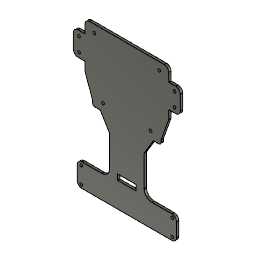
chassis (Autodesk Fusion 360 design; units mm, degrees)
part number: 2026-02-12-20-41-27-995
Autodesk Fusion 360 part; units mm, degrees
sketch "Sketch1" plane through (0, 0, 0) normal (0, 1, 0) x (1, 0, 0)
  line L0 (48.5, 0) -> (-48.5, 0)
  line L1 (-54.5, 6) -> (-54.5, 17)
  line L2 (54.5, 6) -> (54.5, 17)
  line L3 (54.5, 17) -> (54.5, 48) construction
  line L4 (-54.5, 48) -> (-54.5, 59)
  line L5 (54.5, 48) -> (54.5, 59)
  line L6 (54.4997, 87) -> (44.4997, 86.9972) construction
  line L7 (-54.5, 59) -> (-44.4997, 86.9972)
  line L8 (54.5, 59) -> (44.4997, 86.9972)
  line L9 (44.4997, 86.9972) -> (44.4989, 89.9972)
  line L10 (-44.4989, 89.9972) -> (-44.4997, 86.9972)
  line L11 (-41.498, 92.9963) -> (-34.498, 92.9943)
  line L12 (41.498, 92.9963) -> (34.498, 92.9943)
  line L13 (-34.498, 92.9943) -> (-22.5008, 113)
  line L14 (22.5008, 113) -> (34.498, 92.9943)
  line L15 (-22.5008, 113) -> (-22.5122, 153)
  line L16 (22.5008, 113) -> (22.5122, 153)
  line L17 (-32.515, 162.9972) -> (-58.515, 162.9898)
  line L18 (32.515, 162.9972) -> (58.515, 162.9898)
  line L19 (-64.5167, 168.9881) -> (-64.5219, 186.9864)
  line L20 (64.5167, 168.9881) -> (64.5219, 186.9864)
  line L21 (-58.5219, 192.9881) -> (58.5219, 192.9881)
  line L22 (-54.5, 17) -> (-63.5, 17)
  line L23 (-54.5, 48) -> (-63.5, 48)
  line L24 (-69.5, 23) -> (-69.5, 42)
  line L25 (54.5, 17) -> (63.5, 17)
  line L26 (54.5, 48) -> (63.5, 48)
  line L27 (69.5, 42) -> (69.5, 23)
  line L28 (-54.5, 0) -> (-42.1, 0) construction
  line L29 (54.5, 0) -> (42.1, 0) construction
  line L30 (54.5, 10) -> (54.5, 0) construction
  circle A0 centre (-42.1, 10) radius 1.75
  circle A1 centre (42.1, 10) radius 1.75
  circle A2 centre (-30.84, 83.28) radius 1.75
  circle A3 centre (30.84, 83.28) radius 1.75
  circle A4 centre (-62, 23.475) radius 1.75
  circle A5 centre (-62, 41.525) radius 1.75
  circle A6 centre (62, 23.475) radius 1.75
  circle A7 centre (62, 41.525) radius 1.75
  arc A8 (-54.5, 6) -> (-48.5, 0) centre (-48.5, 6) ccw
  arc A9 (48.5, 0) -> (54.5, 6) centre (48.5, 6) ccw
  arc A10 (63.5, 17) -> (69.5, 23) centre (63.5, 23) ccw
  arc A11 (69.5, 42) -> (63.5, 48) centre (63.5, 42) ccw
  arc A12 (-69.5, 23) -> (-63.5, 17) centre (-63.5, 23) ccw
  arc A13 (-63.5, 48) -> (-69.5, 42) centre (-63.5, 42) ccw
  arc A14 (-64.5167, 168.9881) -> (-58.515, 162.9898) centre (-58.5167, 168.9898) ccw
  arc A15 (-58.5219, 192.9881) -> (-64.5219, 186.9864) centre (-58.5219, 186.9881) ccw
  arc A16 (58.515, 162.9898) -> (64.5167, 168.9881) centre (58.5167, 168.9898) ccw
  arc A17 (64.5219, 186.9864) -> (58.5219, 192.9881) centre (58.5219, 186.9881) ccw
  arc A18 (-22.5122, 153) -> (-32.515, 162.9972) centre (-32.5122, 152.9972) ccw
  arc A19 (32.515, 162.9972) -> (22.5122, 153) centre (32.5122, 152.9972) ccw
  arc A20 (44.4989, 89.9972) -> (41.498, 92.9963) centre (41.4989, 89.9963) ccw
  arc A21 (-41.498, 92.9963) -> (-44.4989, 89.9972) centre (-41.4989, 89.9963) ccw
  circle A22 centre (-59.0242, 167.2381) radius 1.75
  circle A23 centre (-59.0327, 188.7381) radius 1.75
  circle A24 centre (59.0242, 167.2381) radius 1.75
  circle A25 centre (59.0327, 188.7381) radius 1.75
  line L31 (-12, 160.5) -> (12, 160.5)
  line L32 (12, 160.5) -> (12, 153.5)
  line L33 (12, 153.5) -> (-12, 153.5)
  line L34 (-12, 153.5) -> (-12, 160.5)
  line L35 (0, -40) -> (0, 250) construction
  point P0 (-38.955, 10.36)
  point P1 (34.555, 10.36)
  point P2 (87.5597, 0)
  point P3 (44.498, 92.9972)
  point P4 (-44.498, 92.9972)
  point P5 (22.515, 163)
  point P6 (-64.515, 162.9881)
  point P7 (64.515, 162.9881)
  point P8 (-64.5236, 192.9881)
  point P9 (64.5236, 192.9881)
  dimension "d154" = 109
  dimension "d155" = 17
  dimension "d156" = 17
  dimension "d167" = 31
  dimension "d168" = 31
  dimension "d177" = 11
  dimension "d178" = 11
  dimension "d180" = 28
  dimension "d182" = 10
  dimension "d184" = 6
  dimension "d191" = 10
  dimension "d192" = 10
  dimension "d194" = 50
  dimension "d196" = 42
  dimension "d197" = 30
  dimension "d198" = 30
  dimension "d203" = 12.4
  dimension "d205" = 12.4
  dimension "d206" = 10
  dimension "d207" = 3.5
  dimension "d208" = 3.5
  dimension "d213" = 3.5
  dimension "d214" = 3.5
  dimension "d221" = 3.5
  dimension "d222" = 3.5
  dimension "d227" = 3.5
  dimension "d228" = 3.5
  dimension "d229" = 6
  dimension "d230" = 6
  dimension "d231" = 6
  dimension "d232" = 6
  dimension "d233" = 6
  dimension "d234" = 6
  dimension "d235" = 6
  dimension "d236" = 6
  dimension "d237" = 6
  dimension "d238" = 6
  dimension "d239" = 10
  dimension "d240" = 10
  dimension "d241" = 3
  dimension "d242" = 3
  dimension "d252" = 3.5
  dimension "d253" = 3.5
  dimension "d254" = 3.5
  dimension "d255" = 3.5
  dimension "d256" = 139
  dimension "d259" = 7
  dimension "d260" = 17.9983
  dimension "d261" = 192.9881
  dimension "d262" = 0.016
  dimension "d263" = 153.5
  dimension "d264" = 4.2484
  dimension "d265" = 25.75
  dimension "d266" = 4.25
  dimension "d267" = 25.7484
  dimension "d268" = 83.28
  dimension "d269" = 9.7133
  dimension "d270" = 10
  dimension "d271" = 82.9965
  dimension "d272" = 23.475
  dimension "d273" = 7.5
  dimension "d274" = 41.525
  dimension "d275" = 7.5
  dimension "d276" = 23.475
  dimension "d277" = 69.5271
  constraint horizontal L0
  constraint coincident origin L0
  constraint perpendicular L0 L1
  constraint perpendicular L0 L2
  constraint parallel L2 L3
  constraint parallel L3 L5
  constraint perpendicular L6 L9
  constraint perpendicular L10 L11
  constraint perpendicular L9 L12
  constraint perpendicular L11 L16
  constraint perpendicular L15 L17
  constraint perpendicular L16 L18
  constraint perpendicular L17 L19
  constraint perpendicular L18 L20
  constraint perpendicular L1 L22
  constraint perpendicular L2 L25
  constraint perpendicular L5 L26
  constraint horizontal L28
  constraint horizontal L29
  constraint vertical L30
  constraint coincident L0 L28.start
  constraint coincident L28.start L1
  constraint tangent L0 A8
  constraint tangent L1 A8
  constraint coincident L0 L29.start
  constraint coincident L29.start L2
  constraint tangent L0 A9
  constraint tangent L2 A9
  constraint tangent L25 A10
  constraint tangent L27 A10
  constraint tangent L26 A11
  constraint tangent L27 A11
  constraint tangent L22 A12
  constraint tangent L24 A12
  constraint tangent L24 A13
  constraint tangent L23 A13
  constraint coincident P6 L17
  constraint coincident P6 L19
  constraint tangent L17 A14
  constraint tangent L19 A14
  constraint coincident P8 L19
  constraint coincident P8 L21
  constraint tangent L19 A15
  constraint tangent L21 A15
  constraint coincident P7 L18
  constraint coincident P7 L20
  constraint tangent L18 A16
  constraint tangent L20 A16
  constraint coincident P9 L21
  constraint coincident P9 L20
  constraint tangent L21 A17
  constraint tangent L20 A17
  constraint tangent L15 A18
  constraint tangent L17 A18
  constraint coincident P5 L16
  constraint coincident P5 L18
  constraint tangent L16 A19
  constraint tangent L18 A19
  constraint coincident P3 L12
  constraint coincident P3 L9
  constraint tangent L12 A20
  constraint tangent L9 A20
  constraint coincident P4 L10
  constraint coincident P4 L11
  constraint tangent L10 A21
  constraint tangent L11 A21
  constraint horizontal L31
  constraint vertical L32
  constraint horizontal L33
  constraint vertical L34
  constraint symmetric L1 L2 L35
  constraint symmetric A8 A9 L35
  constraint symmetric L24 L27 L35
  constraint symmetric L7 L8 L35
  constraint symmetric L4 L5 L35
  constraint symmetric L23 L26 L35
  constraint symmetric A11 A13 L35
  constraint symmetric A10 A12 L35
  constraint symmetric L11 L12 L35
  constraint symmetric L13 L14 L35
  constraint symmetric L15 L16 L35
  constraint symmetric L17 L18 L35
  constraint symmetric A18 A19 L35
  constraint symmetric L19 L20 L35
  constraint symmetric A14 A16 L35
  constraint symmetric A15 A17 L35
  constraint symmetric A22.centre A24.centre L35
  constraint symmetric A23.centre A25.centre L35
  constraint symmetric A0.centre A1.centre L35
  constraint symmetric A5.centre A7.centre L35
  constraint symmetric A2.centre A3.centre L35
  constraint symmetric L32 L34 L35
  measures "d154" distance of L28.start L29.start
  measures "d155" distance of L28.start L1.end
  measures "d156" distance of L29.start L2.end
  measures "d167" distance of L1.end L4.start
  measures "d168" distance of L2.end L3.end
  measures "d177" distance of L4.start L4.end
  measures "d178" distance of L3.end L5.end
  measures "d180" distance of L5.end L6.start
  measures "d182" distance of L6.start L6.end
  measures "d184" distance of L6.end P3
  measures "d191" distance of P4 L11.end
  measures "d192" distance of P3 L12.end
  measures "d194" distance of L14.start P5
  measures "d196" distance of P5 P7
  measures "d197" distance of P6 P8
  measures "d198" distance of P7 P9
  measures "d203" distance of L28.start L28.end
  measures "d205" distance of L29.start L29.end
  measures "d206" distance of L29.start L30.start
  measures "d207" diameter of A0
  measures "d208" diameter of A1
  measures "d213" diameter of A2
  measures "d214" diameter of A3
  measures "d221" diameter of A4
  measures "d222" diameter of A5
  measures "d227" diameter of A6
  measures "d228" diameter of A7
  measures "d229" radius of A8
  measures "d230" radius of A9
  measures "d231" radius of A10
  measures "d232" radius of A11
  measures "d233" radius of A12
  measures "d234" radius of A13
  measures "d235" radius of A14
  measures "d236" radius of A15
  measures "d237" radius of A16
  measures "d238" radius of A17
  measures "d239" radius of A18
  measures "d240" radius of A19
  measures "d241" radius of A20
  measures "d242" radius of A21
  measures "d252" diameter of A22
  measures "d253" diameter of A23
  measures "d254" diameter of A24
  measures "d255" diameter of A25
  measures "d256" distance of L24 L27
  measures "d259" distance of L31.start L33.end
  measures "d260" vertical distance of L19.start L19.end
  measures "d261" distance of L0 L21
  measures "d262" angle of L0 L12
  measures "d263" distance of L0 L33
  measures "d264" distance of L18 A24.centre
  measures "d265" distance of L21 A24.centre
  measures "d266" distance of L21 A25.centre
  measures "d267" distance of L18 A25.centre
  measures "d268" distance of L0 A3.centre
  measures "d269" distance of L12 A3.centre
  measures "d270" distance of L0 A1.centre
  measures "d271" distance of L12 A1.centre
  measures "d272" distance of L0 A6.centre
  measures "d273" distance of L27 A6.centre
  measures "d274" distance of L0 A7.centre
  measures "d275" distance of L27 A7.centre
  measures "d276" distance of L0 A4.centre
  measures "d277" distance of L11 A4.centre
extrude "Extrude1" add sketch "Sketch1" along normal blind 3.1
